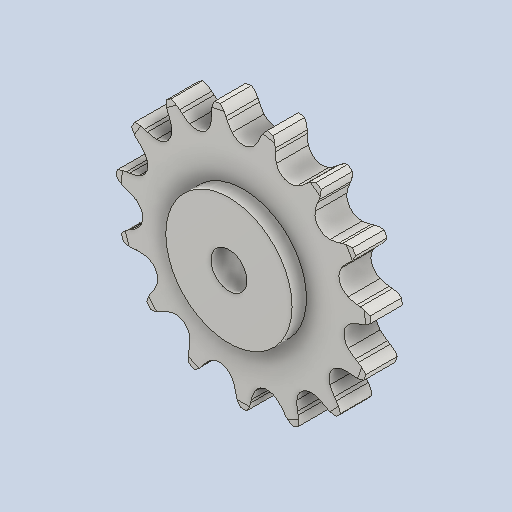
# Autodesk Inventor part: Roller Chain Sprocket1
Saved by Autodesk Inventor 2023 (Build 270158000, 158)
## iProperties
CustomPartVersion: 1
Created: 2023-09-03
Part Number: Roller Chain Sprocket1
Material: Steel
Document SubType Name: Modeling
Designer: sigit
Density: 1 g/cm^3
Appearance: Steel
d28: 0,000 mm
d29: 0,000 mm
d42: 0,000 mm
Author: sigit
Autodesk Inventor part; units mm, degrees
ref_plane "YZ Plane" through (0, 0, 0) normal (1, 0, 0) x (0, 1, 0)
ref_plane "XZ Plane" through (0, 0, 0) normal (0, 1, 0) x (-1, 0, 0)
ref_plane "XY Plane" through (0, 0, 0) normal (0, 0, 1) x (1, 0, 0)
sketch "Theoretical Tooth Profile" plane through (0, 0, 0) normal (0, 0, 1) x (1, 0, 0)
  circle A0 centre (0, 0) radius 19.2389 construction
  line L0 (0, 0) -> (0, 19.2389) construction
  line L1 (0, 0) -> (7.8252, 17.5756) construction
  circle A1 centre (0, 0) radius 21.2185
  arc A2 (-1.872, 17.723) -> (1.872, 17.723) centre (0, 19.2389) ccw
  line L2 (0, 19.2389) -> (7.8252, 17.5756) construction
  line L3 (0, 19.2389) -> (2.9656, 21.6404) construction
  line L4 (2.9656, 21.6404) -> (-2.6882, 19.036) construction
  arc A3 (3.9108, 20.855) -> (2.9106, 19.5187) centre (6.5321, 17.8505) ccw
  arc A4 (-2.9106, 19.5187) -> (-3.9108, 20.855) centre (-6.5321, 17.8505) ccw
  line L5 (-6.5321, 17.8505) -> (-2.9106, 19.5187) construction
  arc A5 (-2.6882, 19.036) -> (-1.872, 17.723) centre (2.9656, 21.6404) ccw
  line L6 (-2.6882, 19.036) -> (-2.9106, 19.5187)
  arc A6 (1.872, 17.723) -> (2.6882, 19.036) centre (-2.9656, 21.6404) ccw
  line L7 (2.9106, 19.5187) -> (2.6882, 19.036)
  line L8 (0, 0) -> (4.4116, 20.7548) construction
  point P0 (3.9126, 18.4073)
  dimension "d0" = 38.4779
  dimension "d2" = 24
  dimension "d3" = 2.4089
  dimension "d10" = 129
  dimension "d11" = 14.267
  dimension "d12" = 3.816
  dimension "d13" = 6.2248
  dimension "d14" = 6.678
  dimension "d23" = 2.4
  constraints: 18 end point, 15 point on circle, 7 centre point, 3 coincident, 3 point on line, 3 symmetric about line, 3 tangent, 1 equal radius, 1 midpoint, 1 parallel, 1 vertical, 1 other
  measures "d0" diameter of A0
  measures "d2" angle of L1 L0
  measures "d3" radius of A2
  measures "d10" angle of L3 L0
  measures "d11" angle of L4 L3
  measures "d12" distance of L2.start L3.end
  measures "d13" distance of L3.end L4.end
  measures "d14" distance of A3.centre L0.end
  measures "d23" distance from line of L8.end L2
sketch "Tooth Profile" plane through (0, 0, 0) normal (0, 0, 1) x (1, 0, 0)
  arc A0 (-2.2174, 18.2977) -> (2.2174, 18.2977) centre (0, 19.2389) ccw
  arc A1 (3.8234, 20.8712) -> (2.2174, 18.2977) centre (11.1746, 14.4956) ccw
  arc A2 (-2.2174, 18.2977) -> (-3.8234, 20.8712) centre (-11.1746, 14.4956) ccw
  line L0 (0, 0) -> (0, 19.2389) construction
  line L1 (0, 19.2389) -> (2.2174, 18.2977) construction
  line L2 (0, 19.2389) -> (-2.2174, 18.2977) construction
  circle A3 centre (0, 0) radius 21.2185 projected
  dimension "d44" = 134
  dimension "d45" = 9.7308
  dimension "d46" = 2.4089
  constraints: 9 point on circle, 6 end point, 3 centre point, 2 tangent, 1 coincident, 1 equal radius, 1 vertical, 1 other
  measures "d44" angle of L2 L1
  measures "d45" radius of A1
  measures "d46" radius of A0
sketch "Section Profile" plane through (0, 0, 0) normal (1, 0, 0) x (0, 1, 0)
  line L0 (21.2185, 0) -> (-21.2185, 0) projected
  line L1 (10.7465, 2.6598) -> (-10.7465, 2.6598)
  line L2 (-10.7465, 2.6598) -> (-10.7465, -2.6598)
  line L3 (-10.7465, -2.6598) -> (10.7465, -2.6598)
  line L4 (10.7465, -2.6598) -> (10.7465, 2.6598)
  line L5 (10.7465, 2.6598) -> (21.2185, 2.6598) construction
  line L6 (21.2185, 2.6598) -> (21.2185, -2.6598) construction
  line L7 (21.2185, -2.6598) -> (10.7465, -2.6598) construction
  line L8 (10.7465, -2.6598) -> (10.7465, 2.6598)
  arc A0 (21.2185, 2.6118) -> (20.3435, 2.6598) centre (20.3435, -5.3402) ccw
  arc A1 (20.3435, -2.6598) -> (21.2185, -2.6118) centre (20.3435, 5.3402) ccw
  line L9 (20.3435, 2.6598) -> (0, 2.6598)
  line L10 (0, 2.6598) -> (0, -2.6598)
  line L11 (0, -2.6598) -> (20.3435, -2.6598)
  line L12 (0, 2.6598) -> (0, -2.6598)
  line L13 (21.2185, 2.6118) -> (21.2185, -2.6118)
  point P0 (0, 0)
  point P1 (0, 0)
  dimension "d30" = 5.3196
  dimension "d31" = 21.493
  dimension "d32" = 5.3196
  dimension "d33" = 0.048
  dimension "d34" = 8
  dimension "d43" = 2.6598
  constraints: 26 end point, 7 midpoint, 5 perpendicular, 4 parallel, 4 point on circle, 3 point on line, 3 symmetric about line, 2 centre point, 2 horizontal, 2 tangent, 1 collinear, 1 other
  measures "d30" distance between parallel lines of L7 L5
  measures "d31" distance between parallel lines of L2 L4
  measures "d32" distance between parallel lines of L3 L1
  measures "d33" distance from line of L13.start L5
  measures "d34" radius of A0
  measures "d43" distance between parallel lines of L3 L0
revolve "Shroud" add sketch "Section Profile" angle 360 about axis through (0, 0, 2.6598) along (0, 0, -1) contours L10 L3 L2 L0 | L0 L2 L1 L10
revolve "Strand" add sketch "Section Profile" angle 360 about axis through (0, 0, 2.6598) along (0, 0, -1) contours L13 A1 L11 L4 L0 | L0 L4 L9 A0 L13 | L4 L3 L10 L0 | L0 L10 L1 L4
pattern_of_one "Strand Pattern"
extrude "Theoretical Tooth" cut sketch "Theoretical Tooth Profile" along normal through all both and the other way through all contours A3 L7 A6 A2 A5 L6 A4 A1 picked at (0, 19.7287)
extrude "Tooth" [suppressed]
pattern_circular "Tooth Pattern" count 15 over 360 about axis through (0, 0, -10) along (0, 0, 1) of "Theoretical Tooth"
ref_plane "Timing Plane" through (0, 19.2389, 0) normal (1, 0, 0) x (0, 1, 0)
sketch "Sketch4" plane through (0, 19.2389, 2.6598) normal (0, 0, 1) x (1, 0, 0)
  circle A0 centre (0, -19.2389) radius 10.5
  dimension "d51" = 21
  constraints: 1 centre point, 1 coincident
  measures "d51" diameter of A0
extrude "Extrusion4" add sketch "Sketch4" along normal blind 2.4
sketch "Sketch5" plane through (0, 19.2389, -2.6598) normal (0, 0, -1) x (-1, 0, 0)
  circle A0 centre (0, -19.2389) radius 10.5
  dimension "d54" = 21
  constraints: 1 centre point, 1 coincident
  measures "d54" diameter of A0
extrude "Extrusion5" add sketch "Sketch5" along normal blind 1.28
sketch "Sketch6" plane through (0, 0, 5.0598) normal (0, 0, 1) x (1, 0, 0)
  circle A0 centre (0, 0) radius 3
  dimension "d57" = 6
  constraints: 1 centre point, 1 coincident
  measures "d57" diameter of A0
extrude "Extrusion6" cut sketch "Sketch6" against normal through all
equation "\"d3\" = 0.5 * da_Dr + da_SC"
equation "\"d12\" = 0.8 * da_Dr"
equation "\"d13\" = 1.3 * da_Dr + da_SC"
equation "\"d14\" = 1.4 * da_Dr"
equation "\"d23\" = da_Ha"
equation "\"d44\" = da_Alfa"
equation "\"d45\" = da_Re"
equation "\"d46\" = da_Ri"
equation "\"d30\" = da_Bf"
equation "\"d31\" = da_Ds"
equation "\"d32\" = da_Bs"
equation "\"d33\" = da_Ba"
equation "\"d34\" = da_Rx"
equation "\"d40\" = da_pt"
equation "\"form_type\" = 0"
equation "\"da_p\" = 8"
equation "\"da_Dr\" = 4.77"
equation "\"da_SC\" = 0.02385"
equation "\"da_Ha\" = 2.4"
equation "\"da_pt\" = 11.6"
equation "\"da_Bf\" = 5.3196"
equation "\"da_Ba\" = 0.048"
equation "\"da_Rx\" = 8"
equation "\"da_Ra\" = 0.32"
equation "\"da_Bs\" = 5.3196"
equation "\"da_Ds\" = 21.49304"
equation "\"da_Re\" = 9.7308"
equation "\"da_Ri\" = 2.40885"
equation "\"da_Alfa\" = 134deg"
body "Solid1"
